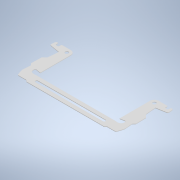
# Autodesk Inventor part: petal_forPrint
Saved by Autodesk Inventor 2022 (Build 260153000, 153)
## iProperties
Created: 2024-12-12
Part Number: petal_forPrint
Material: Типовые
Document SubType Name: Modeling
Designer: Andrey
Density: 1 g/cm^3
Appearance: По умолчанию
Author: Andrey
Autodesk Inventor part; units mm, degrees
ref_plane "YZ Plane" through (0, 0, 0) normal (1, 0, 0) x (0, 1, 0)
ref_plane "XZ Plane" through (0, 0, 0) normal (0, 1, 0) x (-1, 0, 0)
ref_plane "XY Plane" through (0, 0, 0) normal (0, 0, 1) x (1, 0, 0)
sketch "Эскиз1" plane through (0, 0, 0) normal (0, 1, 0) x (-1, 0, 0)
  circle A0 centre (-4.631, -43.5563) radius 1.6
  arc A1 (5, -3.75) -> (5, -6.25) centre (5, -5) ccw
  line L0 (5, -3.75) -> (70, -3.75)
  arc A2 (70, -6.25) -> (70, -3.75) centre (70, -5) ccw
  line L1 (70, -6.25) -> (5, -6.25)
  arc A3 (77.3239, -9.8413) -> (76.131, -9.9442) centre (79.631, -43.5563) ccw
  arc A4 (79.4677, -10.1658) -> (77.3239, -9.8413) centre (77.6653, -14.8296) ccw
  arc A5 (80.6854, -14.8912) -> (79.4677, -10.1658) centre (78.3862, -12.9641) ccw
  line L2 (80.6854, -14.8912) -> (75.8657, -14.0414)
  arc A6 (75.8657, -14.0414) -> (75.631, -14.2384) centre (75.831, -14.2384) ccw
  line L3 (75.631, -14.2384) -> (75.631, -43.5563)
  arc A7 (75.631, -43.5563) -> (79.631, -47.5563) centre (79.631, -43.5563) ccw
  line L4 (79.631, -47.5563) -> (87.8552, -47.5563)
  arc A8 (87.8552, -47.5563) -> (88.6552, -46.7563) centre (87.8552, -46.7563) ccw
  line L5 (88.6552, -46.7563) -> (88.6552, -45.3563)
  arc A9 (89.4552, -44.5563) -> (88.6552, -45.3563) centre (89.4552, -45.3563) ccw
  line L6 (89.4552, -44.5563) -> (90.8552, -44.5563)
  arc A10 (91.6552, -45.3563) -> (90.8552, -44.5563) centre (90.8552, -45.3563) ccw
  line L7 (91.6552, -45.3563) -> (91.6552, -46.7563)
  arc A11 (91.6552, -46.7563) -> (92.4552, -47.5563) centre (92.4552, -46.7563) ccw
  line L8 (92.4552, -47.5563) -> (92.8552, -47.5563)
  arc A12 (92.8552, -47.5563) -> (93.8304, -46.7775) centre (92.8552, -46.5563) ccw
  arc A13 (93.8304, -46.7775) -> (94.174, -42.8497) centre (79.631, -43.5563) ccw
  arc A14 (94.174, -42.8497) -> (93.3489, -41.9134) centre (93.1752, -42.8982) ccw
  line L9 (93.3489, -41.9134) -> (83.9409, -40.2546)
  line L10 (83.9409, -40.2546) -> (84.7989, -30.6198)
  arc A15 (85.1049, -29.9847) -> (84.7989, -30.6198) centre (85.795, -30.7085) ccw
  line L11 (85.1049, -29.9847) -> (87.4169, -27.7806)
  arc A16 (87.4169, -27.7806) -> (87.7266, -27.0807) centre (86.7269, -27.0568) ccw
  line L12 (87.7266, -27.0807) -> (87.9456, -17.9117)
  arc A17 (87.9456, -17.9117) -> (87.6697, -17.1978) centre (86.9459, -17.8878) ccw
  line L13 (87.6697, -17.1978) -> (86.4498, -15.9183)
  arc A18 (86.1776, -15.1396) -> (86.4498, -15.9183) centre (87.1736, -15.2283) ccw
  line L14 (86.1776, -15.1396) -> (86.7309, -8.9267)
  arc A19 (86.7309, -8.9267) -> (86.6462, -7.4668) centre (81.7506, -8.4832) ccw
  arc A20 (86.6462, -7.4668) -> (86.0376, -5.2239) centre (67.7491, -11.39) ccw
  line L15 (86.0376, -5.2239) -> (84.9746, -2.0709)
  arc A21 (84.9746, -2.0709) -> (84.1332, -1.396) centre (84.027, -2.3904) ccw
  arc A22 (84.1332, -1.396) -> (83.7286, -1.3548) centre (79.631, -43.5563) ccw
  arc A23 (83.7286, -1.3548) -> (83.5353, -1.3454) centre (83.5353, -3.3454) ccw
  line L16 (83.5353, -1.3454) -> (76.131, -1.3454)
  line L17 (76.131, -1.3454) -> (75, 0)
  line L18 (0, 0) -> (75, 0)
  line L19 (-1.131, -1.3454) -> (0, 0)
  line L20 (-8.5353, -1.3454) -> (-1.131, -1.3454)
  arc A24 (-8.5353, -1.3454) -> (-8.7286, -1.3548) centre (-8.5353, -3.3454) ccw
  arc A25 (-8.7286, -1.3548) -> (-9.1332, -1.396) centre (-4.631, -43.5563) ccw
  arc A26 (-9.1332, -1.396) -> (-9.9746, -2.0709) centre (-9.027, -2.3904) ccw
  line L21 (-11.0376, -5.2239) -> (-9.9746, -2.0709)
  arc A27 (-11.0376, -5.2239) -> (-11.6462, -7.4668) centre (7.2509, -11.39) ccw
  arc A28 (-11.6462, -7.4668) -> (-11.7309, -8.9267) centre (-6.7506, -8.4832) ccw
  line L22 (-11.1776, -15.1396) -> (-11.7309, -8.9267)
  arc A29 (-11.4498, -15.9183) -> (-11.1776, -15.1396) centre (-12.1736, -15.2283) ccw
  line L23 (-12.6697, -17.1978) -> (-11.4498, -15.9183)
  arc A30 (-12.6697, -17.1978) -> (-12.9456, -17.9117) centre (-11.9459, -17.8878) ccw
  line L24 (-12.7266, -27.0807) -> (-12.9456, -17.9117)
  arc A31 (-12.7266, -27.0807) -> (-12.4169, -27.7806) centre (-11.7269, -27.0568) ccw
  line L25 (-10.1049, -29.9847) -> (-12.4169, -27.7806)
  arc A32 (-9.7989, -30.6198) -> (-10.1049, -29.9847) centre (-10.795, -30.7085) ccw
  line L26 (-8.9409, -40.2546) -> (-9.7989, -30.6198)
  line L27 (-18.3489, -41.9134) -> (-8.9409, -40.2546)
  arc A33 (-18.3489, -41.9134) -> (-19.174, -42.8497) centre (-18.1752, -42.8982) ccw
  arc A34 (-19.174, -42.8497) -> (-18.8304, -46.7775) centre (-4.631, -43.5563) ccw
  arc A35 (-18.8304, -46.7775) -> (-17.8552, -47.5563) centre (-17.8552, -46.5563) ccw
  line L28 (-17.4552, -47.5563) -> (-17.8552, -47.5563)
  arc A36 (-17.4552, -47.5563) -> (-16.6552, -46.7563) centre (-17.4552, -46.7563) ccw
  line L29 (-16.6552, -45.3563) -> (-16.6552, -46.7563)
  arc A37 (-15.8552, -44.5563) -> (-16.6552, -45.3563) centre (-15.8552, -45.3563) ccw
  line L30 (-14.4552, -44.5563) -> (-15.8552, -44.5563)
  arc A38 (-13.6552, -45.3563) -> (-14.4552, -44.5563) centre (-14.4552, -45.3563) ccw
  line L31 (-13.6552, -46.7563) -> (-13.6552, -45.3563)
  arc A39 (-13.6552, -46.7563) -> (-12.8552, -47.5563) centre (-12.8552, -46.7563) ccw
  line L32 (-4.631, -47.5563) -> (-12.8552, -47.5563)
  arc A40 (-4.631, -47.5563) -> (-0.631, -43.5563) centre (-4.631, -43.5563) ccw
  line L33 (-0.631, -14.2384) -> (-0.631, -43.5563)
  arc A41 (-0.631, -14.2384) -> (-0.8657, -14.0414) centre (-0.831, -14.2384) ccw
  line L34 (-5.6854, -14.8912) -> (-0.8657, -14.0414)
  arc A42 (-4.4677, -10.1658) -> (-5.6854, -14.8912) centre (-3.3862, -12.9641) ccw
  arc A43 (-2.3239, -9.8413) -> (-4.4677, -10.1658) centre (-2.6653, -14.8296) ccw
  arc A44 (-1.131, -9.9442) -> (-2.3239, -9.8413) centre (-4.631, -43.5563) ccw
  line L35 (0, -10) -> (-1.131, -9.9442)
  line L36 (75, -10) -> (0, -10)
  line L37 (75, -10) -> (76.131, -9.9442)
  circle A45 centre (79.631, -43.5563) radius 1.6
  constraints: 88 point on circle, 76 end point, 46 centre point
extrude "Выдавливание1" add sketch "Эскиз1" along normal blind 0.5
